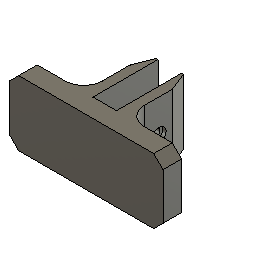
_StopBar.15c0e21f-31c2-4c5c-bdcd-9ff1b70e37b4 (Autodesk Fusion 360 design; units mm, degrees)
Autodesk Fusion 360 part; units mm, degrees
sketch "Sketch1" plane through (0, 0, 0) normal (0, 1, 0) x (1, 0, 0)
  line L0 (16, 0) -> (16, 35)
  line L1 (28.7, 0) -> (28.7, 35)
  line L2 (16, 35) -> (11, 35)
  line L3 (11, 35) -> (11, 0)
  line L4 (16, 0) -> (28.7, 0)
  line L5 (28.7, 35) -> (33.7, 35)
  line L6 (33.7, 35) -> (33.7, 0)
  line L7 (33.7, 0) -> (63.7, 0)
  line L8 (63.7, 0) -> (63.7, -10)
  line L9 (11, 0) -> (-19, 0)
  line L10 (-19, 0) -> (-19, -10)
  line L11 (-19, -10) -> (63.7, -10)
  dimension "d2" = 12.7
  dimension "d3" = 5
  dimension "d4" = 5
  dimension "d5" = 30
  dimension "d6" = 10
  dimension "d7" = 30
  dimension "d8" = 10
  dimension "d16" = 35
  constraint vertical L0
  constraint vertical L1
  constraint perpendicular L0 L2
  constraint perpendicular L2 L3
  constraint perpendicular L1 L4
  constraint perpendicular L1 L5
  constraint perpendicular L5 L6
  constraint perpendicular L6 L7
  constraint perpendicular L7 L8
  constraint perpendicular L3 L9
  constraint perpendicular L9 L10
  constraint perpendicular L8 L11
  constraint horizontal L0.start L3.end
  constraint horizontal L0.end L1.end
  measures "d2" distance of L0 L1
  measures "d3" distance of L0.end L2.end
  measures "d4" distance of L1.end L5.end
  measures "d5" distance of L6.end L7.end
  measures "d6" distance of L7.end L8.end
  measures "d7" distance of L3.end L9.end
  measures "d8" distance of L9.end L10.end
  measures "d16" distance of L2.end L3.end
extrude "Extrude1" add sketch "Sketch1" along normal blind 35
sketch "Sketch2" plane through (33.7, 0, 0) normal (1, 0, 0) x (0, 0, -1)
  line L0 (0, 0) -> (35, 0)
  line L1 (35, 0) -> (35, 35)
  line L2 (35, 35) -> (0, 35)
  line L3 (0, 35) -> (0, 0)
  circle A0 centre (17.9261, 17.0739) radius 2.25
  line L4 (0, 35) -> (16.3351, 18.6649)
  line L5 (19.5171, 15.4829) -> (35, 0)
  line L6 (35, 35) -> (19.0329, 19.0329)
  line L7 (15.9671, 15.9671) -> (0, 0)
  dimension "d11" = 4.5
  constraint coincident L2.end L3.start
  constraint coincident L0.end L1.start
  constraint coincident L1.end L2.start
  constraint coincident L0.start L3.end
  constraint coincident A0 L4.end
  constraint collinear L4 L5
  constraint coincident A0.centre L4
  constraint coincident A0 L5.start
  constraint coincident A0 L6.end
  constraint coincident A0 L7.start
  constraint collinear L6 L7
  measures "d11" diameter of A0
extrude "Extrude2" cut sketch "Sketch2" against normal blind 59 contours A0
ref_plane "WorkPlane1" through (22.35, 17.5, -12.5) normal (0, 1, 0) x (0, 0, 1)
sketch "Sketch3" plane through (0, 17.5, 0) normal (0, 1, 0) x (1, 0, 0)
  line L0 (-20, 0) -> (5, 0)
  line L1 (5, 0) -> (5, -10)
  line L2 (5, -10) -> (-20, -10)
  line L3 (-20, -10) -> (-20, 0)
  line L4 (44, 0) -> (44.05, 0)
  line L5 (33.7, 0) -> (33.7, 35)
  dimension "d14" = 25
  constraint horizontal L0
  constraint vertical L1
  constraint horizontal L2
  constraint vertical L3
  constraint horizontal L4
  measures "d14" distance of L0.start L0.end
sketch "Sketch4" plane through (11, 0, 0) normal (-1, 0, 0) x (0, 0, 1)
  circle A0 centre (-17.9261, 17.0739) radius 2.25 construction
  line L0 (-35, 0) -> (0, 0)
  line L1 (0, 0) -> (0, 35)
  line L2 (0, 35) -> (-35, 35)
  line L3 (-35, 35) -> (-35, 0)
  line L4 (-15.8332, 13.4489) -> (-13.7403, 17.0739)
  line L5 (-13.7403, 17.0739) -> (-15.8332, 20.6989)
  line L6 (-15.8332, 20.6989) -> (-20.019, 20.6989)
  line L7 (-20.019, 20.6989) -> (-22.1119, 17.0739)
  line L8 (-22.1119, 17.0739) -> (-20.019, 13.4489)
  line L9 (-20.019, 13.4489) -> (-15.8332, 13.4489)
  point P0 (-17.9261, 17.0739)
  dimension "d18" = 7.25
  constraint coincident P0 A0.centre
  measures "d18" distance of L6 L9
extrude "Extrude3" cut sketch "Sketch4" against normal blind 3 contours L4 L5 L6 L7 L8 L9
chamfer "Chamfer1" distance 5 angle 45 4 edges at (63.7, 0, 5) (63.7, 35, 5) (-19, 35, 5) (-19, 0, 5)
sketch "Sketch5" plane through (33.7, 0, 0) normal (1, 0, 0) x (0, 0, -1)
  circle A0 centre (17.9261, 17.0739) radius 2.25
  line L0 (0, 0) -> (35, 0)
  line L1 (35, 0) -> (35, 35)
  line L2 (35, 35) -> (0, 35)
  circle A1 centre (17.9261, 17.0739) radius 2.25
  circle A2 centre (17.9261, 17.0739) radius 3.75
  line L3 (0, 35) -> (0, 0)
  dimension "d24" = 7.5
  constraint concentric A1 A2
  measures "d24" diameter of A2
extrude "Extrude4" cut sketch "Sketch5" against normal blind 3.7 contours A2
extrude "Extrude5" cut 1 faces at (14, 18.6077, -15.1575) along direction (1, 0, 0) blind 0.037
extrude "Extrude6" cut 1 faces at (30, 16.7758, -21.1538) along direction (-1, 0, 0) blind 0.663
chamfer "Chamfer2" distance 4 distance2 10 1 edges at (11, 17.5, -35) measured on face at (14.3333, 11.6667, -35)
chamfer "Chamfer2" distance 10 distance2 4 1 edges at (33.7, 17.5, -35) measured on face at (33.7, 30.2711, -17.5486)
extrude "Extrude7" add 1 faces at (14.037, 18.6077, -15.1575) along direction (-1, 0, 0) blind 0.5
extrude "Extrude8" add 1 faces at (29.337, 16.7758, -21.1538) along direction (1, 0, 0) blind 2
extrude "Extrude9" cut 1 faces at (13.537, 18.6077, -15.1575) along direction (1, 0, 0) blind 0.5
extrude "Extrude10" add 1 faces at (31.337, 16.7758, -21.1538) along direction (1, 0, 0) blind 0.5
fillet "Fillet1" radius 10 2 edges at (33.7, 17.5, 0) (11, 17.5, 0)
equation "d5 = d7"
